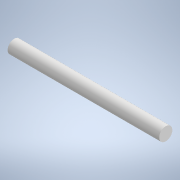
# Autodesk Inventor part: AVI_screw_part1.1
Saved by Autodesk Inventor 2022 (Build 260153000, 153)
## iProperties
Created: 2022-08-03
Part Number: AVI_screw_part1.1
Material: Generic
Document SubType Name: Modeling
Designer: dovalle
Density: 1 g/cm^3
Appearance: Default
Author: dovalle
Autodesk Inventor part; units mm, degrees
ref_plane "YZ Plane" through (0, 0, 0) normal (1, 0, 0) x (0, 1, 0)
ref_plane "XZ Plane" through (0, 0, 0) normal (0, 1, 0) x (-1, 0, 0)
ref_plane "XY Plane" through (0, 0, 0) normal (0, 0, 1) x (1, 0, 0)
sketch "Sketch2" plane through (0, 0, 0) normal (1, 0, 0) x (0, 1, 0)
  circle A0 centre (0, 0) radius 4.35
  dimension "d3" = 8.7
  constraints: 1 centre point, 1 coincident
  measures "d3" diameter of A0
extrude "Extrusion2" add sketch "Sketch2" along normal blind 100
body "Solid2"
